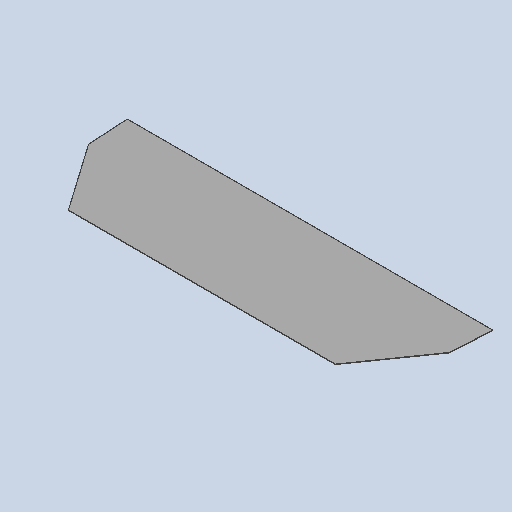
# Autodesk Inventor part: MSC 704 face 4
Saved by Autodesk Inventor 2025 (Build 290162010, 162A)
## iProperties
Created: 2024-06-16
Part Number: MSC 704 face 4
Material: Stainless Steel
Document SubType Name: Sheet Metal
Designer: admin
Density: 8 g/cm^3
Sheet Metal Rule: AISI304 2mm Die16
Appearance: Default
Stock Number: МОО 704 морда 4
Flat Pattern Width: 45 cm
Flat Pattern Length: 151.98 cm
Flat Pattern Area: 6839.1 cm^2
Sheet Metal Width: 450,000 mm
Sheet Metal Length: 1519,800 mm
Sheet Metal Area: 683910,000 mm^2
Mass: 9956.61 g
Surface Area: 12518.8 cm^2
Volume: 1244.58 cm^3
Author: admin
Autodesk Inventor part; units mm, degrees
ref_plane "YZ Plane" through (0, 0, 0) normal (1, 0, 0) x (0, 1, 0)
ref_plane "XZ Plane" through (0, 0, 0) normal (0, 1, 0) x (-1, 0, 0)
ref_plane "XY Plane" through (0, 0, 0) normal (0, 0, 1) x (1, 0, 0)
sketch "Sketch1" plane through (0, 0, 0) normal (0, 0, 1) x (1, 0, 0)
  line L0 (-760, -450) -> (760, -450)
  line L1 (760, -450) -> (760, 0)
  line L2 (760, 0) -> (-760, 0)
  line L3 (-760, 0) -> (-760, -450)
  point P0 (0, 0)
  point P1 (0, 0)
  dimension "d0" = 450
  dimension "d1" = 1520
  measures "d0" distance of L2.end L0.start
  measures "d1" distance of L1.end L2.end
extrude "Plate1" add sketch "Sketch1" along normal blind 2
sketch "Sketch2" plane through (0, 0, 2) normal (0, 0, 1) x (1, 0, 0)
  line L0 (760, -450) -> (-760, -450) projected
  line L1 (760, 0) -> (760, -450) projected
  line L2 (-760, 0) -> (760, 0) projected
  line L3 (-760, -450) -> (-760, 0) projected
  line L4 (759.9, 0) -> (750, -171)
  line L5 (750, -171) -> (555, -450)
  line L6 (760, -450) -> (-760, -450) projected
  point P0 (0, 0)
  dimension "d3" = 0.1
  dimension "d8" = 10
  dimension "d9" = 171
  dimension "d10" = 205
  constraints: 4 end point, 2 point on line
  measures "d3" distance of L1.start L4.start
  measures "d8" distance from line of L1 L4.end
  measures "d9" distance from line of L2 L4.end
  measures "d10" distance of L0.start L5.end
extrude "Extrusion1" cut sketch "Sketch2" against normal through all contours L0 L5 L4 L2 L1
mirror "Mirror1" about plane through (0, 0, 0) normal (1, 0, 0) of "Extrusion1"
equation "\"d2\" = Thickness"
equation "\"BendReliefWidth\" = Thickness"
equation "\"BendReliefDepth\" = 0.5 * Thickness"
equation "\"CornerReliefSize\" = 4 * Thickness"
equation "\"MinimumRemnant\" = 2 * Thickness"
equation "\"TransitionRadius\" = BendRadius"
equation "\"JacobiRadiusSize\" = BendRadius"
equation "\"GapSize\" = Thickness"
equation "\"Thickness\" = 2"
equation "\"BendRadius\" = 2.75"
body "Solid1"
